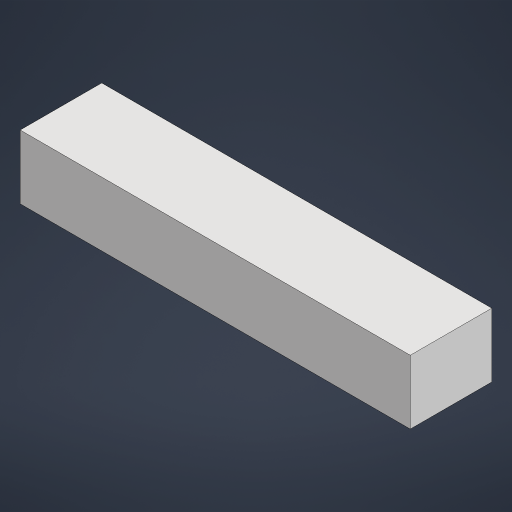
# Autodesk Inventor part: WDW_rtn
Saved by Autodesk Inventor 2023.1 (Build 271208000, 208)
## iProperties
Created: 2022-11-19
Part Number: WDW_rtn
Material: Generic
Document SubType Name: Modeling
Designer: awelt
Mass: 6078.61 g
Surface Area: 2571.57 cm^2
Volume: 6078.61 cm^3
Density: 1 g/cm^3
Appearance: Default
RuleStatus: InUse
BeforeDocSave0: file://C:\Users\awelt\Documents\Inventor\iLogic_Rules\BoundingStore
DocClose0: file://C:\Users\awelt\Documents\Inventor\iLogic_Rules\BoundingStore
Author: awelt
BoundingBL1: 3 5/8
BoundingBL2: 4 5/8
BoundingBL3: 22 1/8
BoundingCF: 0.215
Autodesk Inventor part; units mm, degrees
ref_plane "YZ Plane" through (0, 0, 0) normal (1, 0, 0) x (0, 1, 0)
ref_plane "XZ Plane" through (0, 0, 0) normal (0, 1, 0) x (-1, 0, 0)
ref_plane "XY Plane" through (0, 0, 0) normal (0, 0, 1) x (1, 0, 0)
sketch "Sketch2" plane through (0, 0, 0) normal (0, 1, 0) x (-1, 0, 0)
  line L0 (0, 0) -> (-561.975, 0)
  line L1 (-561.975, 0) -> (-561.975, -117.475)
  line L2 (-561.975, -117.475) -> (0, -117.475)
  line L3 (0, -117.475) -> (0, 0)
  dimension "d3" = 561.975
  dimension "d4" = 117.475
  constraints: 8 end point, 2 parallel, 1 horizontal, 1 perpendicular
  measures "d3" distance of L2.end L1.end
  measures "d4" distance of L1.end L0.end
extrude "Extrusion1" add sketch "Sketch2" along normal blind 92.075
body "Solid1"
